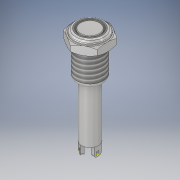
# Autodesk Inventor part: Power Button
Saved by Autodesk Inventor 2019.4 (Build 234330000, 330)
## iProperties
Created: 2018-12-14
Part Number: Power Button
Material: Aluminum 6061-AHC
Document SubType Name: Modeling
Designer: Petar
Density: 2.7 g/cm^3
Appearance: Aluminum - Dark
Mass: 6.0336 g
Surface Area: 10.9701 cm^2
Volume: 2.23467 cm^3
Author: Petar
Autodesk Inventor part; units mm, degrees
ref_plane "YZ Plane" through (0, 0, 0) normal (1, 0, 0) x (0, 1, 0)
ref_plane "XZ Plane" through (0, 0, 0) normal (0, 1, 0) x (-1, 0, 0)
ref_plane "XY Plane" through (0, 0, 0) normal (0, 0, 1) x (1, 0, 0)
sketch "Sketch1" plane through (0, 0, 0) normal (0, 1, 0) x (-1, 0, 0)
  circle A0 centre (0, 0) radius 6.5
  line L0 (7.0179, -4.0102) -> (0.036, -8.0828)
  line L1 (0.036, -8.0828) -> (-6.9819, -4.0726)
  line L2 (-6.9819, -4.0726) -> (-7.0179, 4.0102)
  line L3 (-7.0179, 4.0102) -> (-0.036, 8.0828)
  line L4 (-0.036, 8.0828) -> (6.9819, 4.0726)
  line L5 (6.9819, 4.0726) -> (7.0179, -4.0102)
  circle A1 centre (0, 0) radius 5.5
  dimension "d0" = 13
  dimension "d1" = 14
  dimension "d2" = 11
  constraints: 12 end point, 3 coincident, 2 centre point, 13 other
  measures "d0" diameter of A0
  measures "d1" distance between parallel lines of L2 L5
  measures "d2" diameter of A1
extrude "Extrusion1" add sketch "Sketch1" against normal blind 18 contours A1
extrude "Extrusion2" add sketch "Sketch1" against normal blind 5 contours A0
extrude "Extrusion3" add sketch "Sketch1" against normal blind 5 separate body contours L0 L1 L2 L3 L4 L5
extrude "Extrusion4" cut sketch "Sketch1" against normal blind 1.5 contours L0 L1 L2 L3 L4 L5 bodies 1 2
sketch "Sketch3" plane through (0, 0, 0) normal (0, 0, 1) x (1, 0, 0)
  line L0 (10.5179, 1.8932) -> (10.5179, -8.5662)
  line L1 (7.0179, 0) -> (7.0179, -5) projected
  line L2 (9.5179, -3.25) -> (2.1727, 1.8932)
  line L3 (9.5179, -3.25) -> (2.1727, -3.25) construction
  line L4 (2.1727, -3.25) -> (2.1727, 1.8932) construction
  line L5 (10.5179, 1.8932) -> (2.1727, 1.8932)
  line L6 (10.5179, -8.5662) -> (1.9257, -8.5662)
  line L7 (1.9257, -8.5662) -> (9.5179, -3.25)
  line L8 (0, 0) -> (0, 6) construction
  point P0 (7.0179, -1.5)
  dimension "d25" = 3.5
  dimension "d26" = 1
  dimension "d27" = 35
  dimension "d28" = 35
  constraints: 16 end point, 2 horizontal, 2 perpendicular, 1 vertical
  measures "d25" distance between parallel lines of L0 L1
  measures "d26" distance from line of L0 L2.start
  measures "d27" angle of L3 L2
  measures "d28" angle of L7 L3
chamfer "Chamfer1" distance 1 angle 45 1 edges at (6.5, 0, 0)
fillet "Fillet1" radius 1 1 edges at (5.5, 0, 0)
fillet "Fillet2" radius 2 1 edges at (5.5, -18, 0)
sketch "Sketch2" plane through (0, 0, 0) normal (0, 1, 0) x (1, 0, 0)
  circle A0 centre (0, 0) radius 5.0858 projected
  circle A1 centre (0, 0) radius 4
  dimension "d16" = 8
  constraints: 1 centre point, 1 coincident
  measures "d16" diameter of A1
extrude "Extrusion5" cut sketch "Sketch2" against normal blind 1 contours A1 bodies 1
chamfer "Chamfer2" distance 0.5 angle 45 1 edges at (-4, 0, 0)
extrude "Extrusion6" add sketch "Sketch2" against normal blind 1 contours A1 bodies 1
fillet "Fillet3" radius 0.2 1 edges at (-4, 0, 0)
revolve "Revolution1" cut sketch "Sketch3" angle 360 about axis through (0, 0, 0) along (0, 1, 0) bodies 2 contours L0 L6 L7 L2 L5
combine bodies "Combine1" operation type add bodies to combine 2 1
sketch "Sketch7" plane through (0, -18, 0) normal (0, -1, 0) x (1, 0, 0)
  circle A0 centre (0, 0) radius 3.5 projected
extrude "Extrusion10" add sketch "Sketch7" along normal blind 22 bodies 2
ref_plane "Work Plane1" through (0, -44, 0) normal (0, -1, 0) x (1, 0, 0)
sketch "Sketch4" plane through (0, -44, 0) normal (0, -1, 0) x (1, 0, 0)
  line L0 (3.1623, 1.5) -> (2.1623, 1.5)
  line L1 (2.1623, 1.5) -> (2.1623, -1.5)
  line L2 (2.1623, -1.5) -> (3.1623, -1.5)
  line L3 (3.1623, -1.5) -> (3.1623, 1.5)
  line L4 (0, 0) -> (2.1623, 0) construction
  line L5 (-2.8802, 1.9886) -> (-2.3802, 1.1226)
  line L6 (-2.3802, 1.1226) -> (0.2179, 2.6226)
  line L7 (0.2179, 2.6226) -> (-0.2821, 3.4886)
  line L8 (-0.2821, 3.4886) -> (-2.8802, 1.9886)
  line L9 (-0.2821, -3.4886) -> (0.2179, -2.6226)
  line L10 (0.2179, -2.6226) -> (-2.3802, -1.1226)
  line L11 (-2.3802, -1.1226) -> (-2.8802, -1.9886)
  line L12 (-2.8802, -1.9886) -> (-0.2821, -3.4886)
  circle A0 centre (0, 0) radius 3.5 construction
  point P0 (-1.0811, 1.8726)
  point P1 (-1.0811, -1.8726)
  dimension "d31" = 1
  dimension "d32" = 3
  dimension "d35" = 360
  constraints: 26 end point, 3 midpoint, 2 horizontal, 2 parallel, 1 perpendicular, 31 other
  measures "d31" distance of L1.end L2.end
  measures "d32" distance of L0.end L1.end
extrude "Extrusion7" add sketch "Sketch4" against normal up to next bodies 2
fillet "Fillet4" radius 1 6 edges at (-2.6302, -44, 1.5556) (-0.0321, -44, 3.0556) (2.6623, -44, 1.5) (2.6623, -44, -1.5) (-2.6302, -44, -1.5556) (-0.0321, -44, -3.0556)
sketch "Sketch5" plane through (-0.2821, -43, 3.4886) normal (-0.5, 0, 0.8660254) x (0.8660254, 0, 0.5)
  line L0 (-1, -0.3962) -> (-2, -0.3962)
  line L1 (-2, -0.3962) -> (-2, 0.8038)
  line L2 (-2, 0.8038) -> (-1, 0.8038)
  line L3 (-1, 0.8038) -> (-1, -0.3962)
  line L4 (-1.5, -0.3962) -> (-1.5, 0.8038) construction
  line L5 (-2, 0.2038) -> (-1, 0.2038) construction
  point P0 (-1.5, 43)
  dimension "d40" = 1.2
  constraints: 12 end point, 4 midpoint, 2 parallel, 1 horizontal, 1 perpendicular
  measures "d40" distance of L0.end L1.end
extrude "Extrusion8" cut sketch "Sketch5" against normal up to next bodies 2
pattern_circular "Circular Pattern1" count 3 over 360 about axis through (0, -16, 0) along (0, -1, 0) of "Extrusion8" bodies 2
thread "Thread1" size "M12x1.75" class "6g" standard "ANSI Metric M Profile" full length
chamfer "Chamfer3" distance 0.2 angle 45 1 edges at (6.5, -1, 0)
body "Solid2"
